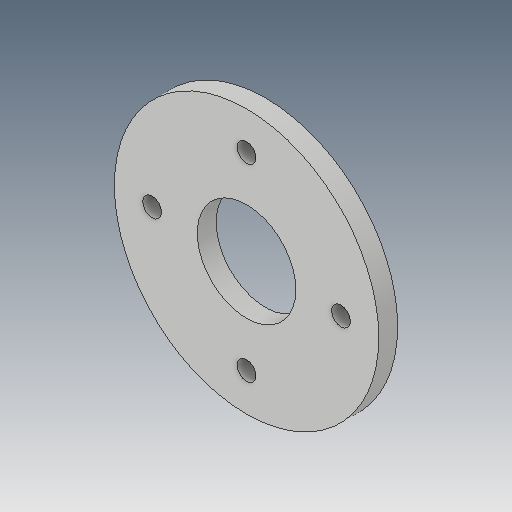
# Autodesk Inventor part: 車軸受け板3
Saved by Autodesk Inventor 2020.3 (Build 243373000, 373)
## iProperties
Part Number: 車軸受け板3
Material: 一般
Document SubType Name: Modeling
Designer: highs
Density: 1 g/cm^3
Appearance: 既定
Stock Number: 要調査
Author: highs
Autodesk Inventor part; units mm, degrees
ref_plane "YZ Plane" through (0, 0, 0) normal (1, 0, 0) x (0, 1, 0)
ref_plane "XZ Plane" through (0, 0, 0) normal (0, 1, 0) x (-1, 0, 0)
ref_plane "XY Plane" through (0, 0, 0) normal (0, 0, 1) x (1, 0, 0)
sketch "スケッチ1" plane through (0, 0, 0) normal (0, 0, 1) x (1, 0, 0)
  circle A0 centre (0, 0) radius 35
  circle A1 centre (0, 0) radius 13.05
  circle A2 centre (0, 0) radius 25 construction
  line L0 (0, 35) -> (0, 0) construction
  line L1 (0, 0) -> (35, 0) construction
  circle A3 centre (25, 0) radius 2.5
  circle A4 centre (0, 25) radius 2.5
  circle A5 centre (-25, 0) radius 2.5
  circle A6 centre (0, -25) radius 2.5
  dimension "d3" = 50
  dimension "d0" = 26.1
  dimension "d1" = 70
  dimension "d2" = 5
  dimension "d6" = 360
  constraints: 6 centre point, 4 end point, 3 coincident, 2 point on circle, 1 horizontal alignment, 1 perpendicular, 1 point on line, 1 vertical, 11 other
  measures "d0" diameter of A1
  measures "d1" diameter of A0
  measures "d2" diameter of A3
extrude "押し出し1" add sketch "スケッチ1" along normal blind 5
